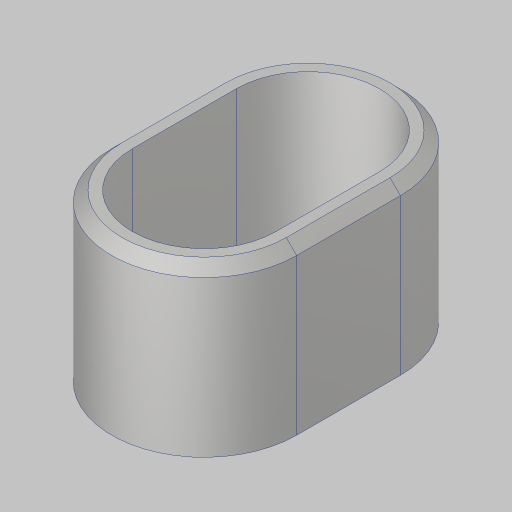
# Autodesk Inventor part: WL-006
Saved by Autodesk Inventor 2023.5 (Build 275446000, 446)
## iProperties
Created: 2025-02-28
Part Number: WL-006
Material: Aluminum 6061
Document SubType Name: Modeling
Designer: slick
Density: 2.7 g/cm^3
Appearance: Aluminum - Flat
Author: slick
Autodesk Inventor part; units mm, degrees
ref_plane "YZ Plane" through (0, 0, 0) normal (1, 0, 0) x (0, 1, 0)
ref_plane "XZ Plane" through (0, 0, 0) normal (0, 1, 0) x (-1, 0, 0)
ref_plane "XY Plane" through (0, 0, 0) normal (0, 0, 1) x (1, 0, 0)
sketch "Sketch1" plane through (0, 0, 0) normal (0, 1, 0) x (-1, 0, 0)
  line L0 (0, -7.9375) -> (0, 7.9375) construction
  line L1 (17.4625, -7.9375) -> (17.4625, 7.9375) construction
  line L2 (-17.4625, 7.9375) -> (-17.4625, -7.9375) construction
  arc A0 (-17.4625, -7.9375) -> (17.4625, -7.9375) centre (0, -7.9375) ccw construction
  arc A1 (17.4625, 7.9375) -> (-17.4625, 7.9375) centre (0, 7.9375) ccw construction
  line L3 (14.1605, 7.9375) -> (14.1605, -7.9375)
  arc A2 (-14.1605, -7.9375) -> (14.1605, -7.9375) centre (0, -7.9375) ccw
  line L4 (-14.1605, -7.9375) -> (-14.1605, 7.9375)
  arc A3 (14.1605, 7.9375) -> (-14.1605, 7.9375) centre (0, 7.9375) ccw
  line L5 (10.9855, -7.9375) -> (10.9855, 7.9375)
  arc A4 (10.9855, 7.9375) -> (-10.9855, 7.9375) centre (0, 7.9375) ccw
  line L6 (-10.9855, 7.9375) -> (-10.9855, -7.9375)
  arc A5 (-10.9855, -7.9375) -> (10.9855, -7.9375) centre (0, -7.9375) ccw
  point P0 (0, 0)
  point P1 (0, 25.4)
  point P2 (0, -25.4)
  dimension "d1" = 34.925
  dimension "d2" = 3.302
  dimension "d3" = 50.8
  dimension "d15" = 3.175
  constraints: 16 end point, 14 point on circle, 6 centre point, 4 tangent, 3 parallel, 1 midpoint, 1 vertical, 6 other
  measures "d1" distance between parallel lines of L2 L1
  measures "d2" distance between parallel lines of L1 L3
  measures "d3" distance of point (0, 25.4) point (0, -25.4)
  measures "d15" radial gap between concentric circles of A2 A5
extrude "Extrusion1" add sketch "Sketch1" along normal mid plane 25.4
chamfer "Chamfer2" distance 1.5875 angle 45 4 edges at (0, 12.7, 22.098) (14.1605, 12.7, 0) (0, 12.7, -22.098) (-14.1605, 12.7, 0)
body "Solid1"
